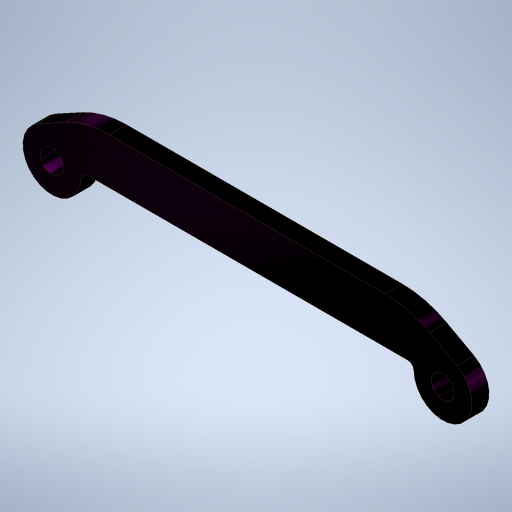
# Autodesk Inventor part: Front Lower Arm Brace
Saved by Autodesk Inventor 2023.1 (Build 271208000, 208)
## iProperties
Created: 2019-11-19
Part Number: Front Lower Arm Brace
Material: Generic
Document SubType Name: Modeling
Designer: Jopa
Density: 1 g/cm^3
Appearance: Brindle
Author: Jopa
Autodesk Inventor part; units mm, degrees
ref_plane "YZ Plane" through (0, 0, 0) normal (1, 0, 0) x (0, 1, 0)
ref_plane "XZ Plane" through (0, 0, 0) normal (0, 1, 0) x (-1, 0, 0)
ref_plane "XY Plane" through (0, 0, 0) normal (0, 0, 1) x (1, 0, 0)
sketch "Sketch1" plane through (0, 0, 0) normal (0, 0, 1) x (1, 0, 0)
  line L0 (-22.225, 0) -> (22.225, 0)
  line L1 (-22.225, 0) -> (-28.8416, -3.6137)
  arc A0 (-28.8416, -3.6137) -> (-22.9235, -7.1247) centre (-26.924, -7.1247) ccw
  line L2 (-22.9235, -7.1247) -> (-22.9235, -6.35)
  circle A1 centre (-26.924, -7.1247) radius 1.5875
  line L3 (0, -15.1277) -> (0, 2.5213) projected
  line L4 (22.225, 0) -> (28.8416, -3.6137)
  arc A2 (22.9235, -7.1247) -> (28.8416, -3.6137) centre (26.924, -7.1247) ccw
  line L5 (22.9235, -7.1247) -> (22.9235, -6.35)
  circle A3 centre (26.924, -7.1247) radius 1.5875
  line L6 (-22.9235, -6.35) -> (22.9235, -6.35)
  point P0 (0, 0)
  point P1 (0, 0)
  point P2 (-26.924, -11.1252)
  point P3 (26.924, -11.1252)
  dimension "d0" = 8.001
  dimension "d1" = 3.175
  dimension "d2" = 4.7752
  dimension "d3" = 6.35
  dimension "d4" = 44.45
  dimension "d5" = 53.848
  constraints: 12 end point, 6 point on circle, 6 symmetric about line, 4 centre point, 3 coincident, 2 horizontal, 2 tangent, 1 midpoint, 1 vertical, 1 vertical alignment, 2 other
  measures "d0" diameter of A0
  measures "d1" diameter of A1
  measures "d2" vertical distance of point (-26.924, -11.125) L2.end
  measures "d3" distance from line of L0 L2.end
  measures "d4" distance of L0.start L0.end
  measures "d5" diameter of A0.centre L3
extrude "Extrusion1" add sketch "Sketch1" along normal mid plane 2.3813
fillet "Fillet1" radius 12.7 2 edges at (-22.225, 0, 0) (22.225, 0, 0)
fillet "Fillet2" radius 0.8128 2 edges at (-22.9235, -6.35, 0) (22.9235, -6.35, 0)
body "Solid1"
